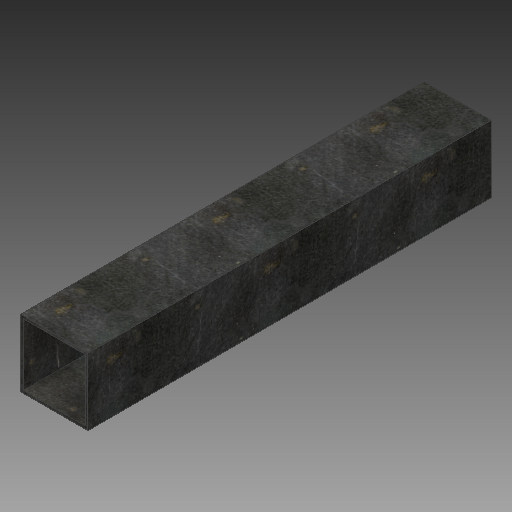
# Autodesk Inventor part: 45 STEEL PROFILE
Saved by Autodesk Inventor 2018 (Build 220112000, 112)
## iProperties
Part Number: 45 STEEL PROFILE
Material: Acero
Document SubType Name: Modeling
Designer: Cristian
Density: 7.85 g/cm^3
Appearance: Placa
Author: Cristian
Autodesk Inventor part; units mm, degrees
ref_plane "YZ Plane" through (0, 0, 0) normal (1, 0, 0) x (0, 1, 0)
ref_plane "XZ Plane" through (0, 0, 0) normal (0, 1, 0) x (-1, 0, 0)
ref_plane "XY Plane" through (0, 0, 0) normal (0, 0, 1) x (1, 0, 0)
sketch "Boceto1" plane through (0, 0, 0) normal (0, 0, 1) x (1, 0, 0)
  line L0 (-37.5, 37.5) -> (37.5, 37.5)
  line L1 (37.5, 37.5) -> (37.5, -37.5)
  line L2 (37.5, -37.5) -> (-37.5, -37.5)
  line L3 (-37.5, -37.5) -> (-37.5, 37.5)
  line L4 (34.5, 34.5) -> (-34.5, 34.5)
  line L5 (-34.5, 34.5) -> (-34.5, -34.5)
  line L6 (-34.5, -34.5) -> (34.5, -34.5)
  line L7 (34.5, -34.5) -> (34.5, 34.5)
  point P0 (0, 0)
  dimension "d0" = 75
  dimension "d1" = 75
  dimension "d2" = 3
  dimension "d3" = 37.5
  dimension "d4" = 37.5
  constraints: 16 end point, 4 parallel, 2 perpendicular, 1 horizontal, 3 other
  measures "d0" distance of L0.start L0.end
  measures "d1" distance of L0.end L1.end
  measures "d2" distance between parallel lines of L0 L4
  measures "d3" distance from line of point (0, 0) L0
  measures "d4" distance from line of point (0, 0) L3
extrude "Extrusión1" add sketch "Boceto1" along normal mid plane 450
equation "\"d0\" = width"
equation "\"d1\" = height"
equation "\"d2\" = t"
equation "\"d3\" = 0.5 * height"
equation "\"d4\" = 0.5 * width"
equation "\"d5\" = length"
equation "\"width\" = 75"
equation "\"height\" = 75"
equation "\"t\" = 3"
equation "\"length\" = 450"
